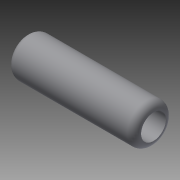
# Autodesk Inventor part: RubberHandleSleeveTL
Saved by Autodesk Inventor 2015 (Build 190159000, 159)
## iProperties
Created: 2015-01-29
Part Number: RubberHandleSleeveTL
Material: Generic
Document SubType Name: Modeling
Designer: PLTW-Stu-02
Density: 1 g/cm^3
Appearance: Default
Author: PLTW-Stu-02
Autodesk Inventor part; units mm, degrees
ref_plane "YZ Plane" through (0, 0, 0) normal (1, 0, 0) x (0, 1, 0)
ref_plane "XZ Plane" through (0, 0, 0) normal (0, 1, 0) x (-1, 0, 0)
ref_plane "XY Plane" through (0, 0, 0) normal (0, 0, 1) x (1, 0, 0)
sketch "Sketch1" plane through (0, 0, 0) normal (0, 0, 1) x (1, 0, 0)
  line L0 (131.6695, 17.9467) -> (18.1569, 17.9467) construction
  line L1 (18.1569, 17.9467) -> (131.6695, 17.9467)
  line L2 (131.6695, 17.9467) -> (131.6695, 24.2967)
  line L3 (131.6695, 24.2967) -> (22.1193, 24.2967)
  line L4 (18.1569, 17.9467) -> (18.1569, 33.0406)
  line L5 (18.1569, 33.0406) -> (22.1193, 33.0406)
  line L6 (22.1193, 33.0406) -> (22.1193, 24.2967)
  line L7 (131.6695, 35.4092) -> (50.1187, 35.4219) construction
  dimension "d3" = 113.5126
  constraints: 16 end point, 2 perpendicular, 1 collinear, 1 vertical
  measures "d3" distance of L0.start L0.end
revolve "Revolution1" add sketch "Sketch1" angle 360 about axis through (131.6695, 35.4092, 0) along (-1, 0.0001557, 0)
fillet "Fillet1" radius 6.35 1 edges at (131.6749, 52.8717, 0)
fillet "Fillet2" radius 6.35 1 edges at (18.1623, 52.9071, 0)
body "Solid1"
